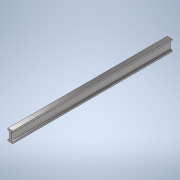
# Autodesk Inventor part: A Console beam
Saved by Autodesk Inventor 2021 (Build 250183000, 183)
## iProperties
Created: 2021-03-20
Part Number: A Console beam
Material: Steel, Cast
Document SubType Name: Modeling
Designer: TieuBinh
Density: 7.85 g/cm^3
Appearance: Semi-Polished
Mass: 69080 g
Surface Area: 9688 cm^2
Volume: 8800 cm^3
Author: TieuBinh
Autodesk Inventor part; units mm, degrees
ref_plane "YZ Plane" through (0, 0, 0) normal (1, 0, 0) x (0, 1, 0)
ref_plane "XZ Plane" through (0, 0, 0) normal (0, 1, 0) x (-1, 0, 0)
ref_plane "XY Plane" through (0, 0, 0) normal (0, 0, 1) x (1, 0, 0)
sketch "Sketch1" plane through (0, 0, 0) normal (0, 0, 1) x (1, 0, 0)
  line L0 (10, 0) -> (10, 50)
  line L1 (10, 50) -> (30, 50)
  line L2 (30, 50) -> (30, 70)
  line L3 (30, 70) -> (0, 70)
  line L4 (10, 0) -> (10, -50)
  line L5 (10, -50) -> (30, -50)
  line L6 (30, -50) -> (30, -70)
  line L7 (30, -70) -> (0, -70)
  line L8 (-10, 0) -> (-10, 50)
  line L9 (-10, 50) -> (-30, 50)
  line L10 (-30, 50) -> (-30, 70)
  line L11 (-30, 70) -> (0, 70)
  line L12 (-10, 0) -> (-10, -50)
  line L13 (-10, -50) -> (-30, -50)
  line L14 (-30, -50) -> (-30, -70)
  line L15 (-30, -70) -> (0, -70)
  point P0 (0, 0)
  dimension "d4" = 50
  dimension "d5" = 20
  dimension "d6" = 20
  constraints: 32 end point, 3 perpendicular
  measures "d4" distance of L0.start L0.end
  measures "d5" distance of L0.end L1.end
  measures "d6" distance of L1.end L2.end
extrude "Extrusion1" add sketch "Sketch1" along normal blind 2000
body "Solid1"
